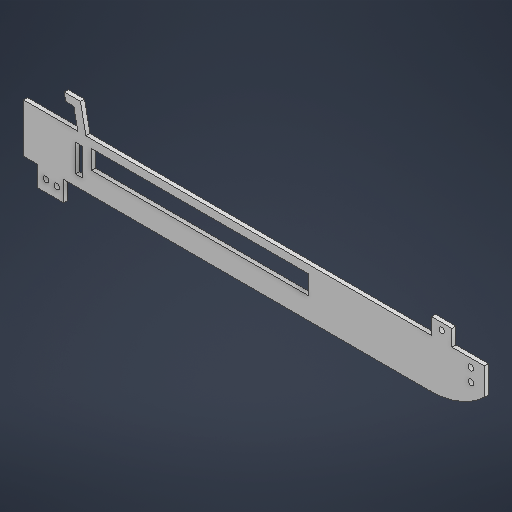
# Autodesk Inventor part: Middle_bar
Saved by Autodesk Inventor 2027 (Build 310192000, 192)
## iProperties
Created: 2026-05-09
Part Number: Middle_bar
Material: Generic
Document SubType Name: Modeling
Designer: alexy
Density: 1 g/cm^3
Appearance: Default
Mass: 26.8499 g
Surface Area: 216.911 cm^2
Volume: 26.8499 cm^3
Author: alexy
Autodesk Inventor part; units mm, degrees
ref_plane "YZ Plane" through (0, 0, 0) normal (1, 0, 0) x (0, 1, 0)
ref_plane "XZ Plane" through (0, 0, 0) normal (0, 1, 0) x (-1, 0, 0)
ref_plane "XY Plane" through (0, 0, 0) normal (0, 0, 1) x (1, 0, 0)
sketch "Sketch1" plane through (0, 0, 0) normal (0, 0, 1) x (1, 0, 0)
  line L0 (0, 0) -> (300, 0)
  line L1 (300, 0) -> (300, 16)
  line L2 (300, 16) -> (0, 16)
  line L3 (0, 16) -> (0, 0)
  line L4 (0, 0) -> (22.0483, 0)
  line L5 (10, 0) -> (29.5, 0)
  line L6 (29.5, 0) -> (29.5, -15)
  line L7 (29.5, -15) -> (10, -15)
  line L8 (10, -15) -> (10, 0)
  point P0 (0, 8)
  dimension "d2" = 19.5
  dimension "d3" = 15
  dimension "d4" = 10
  dimension "d5" = 16
  dimension "d8" = 300
  constraints: 18 end point, 4 parallel, 3 horizontal, 2 perpendicular, 1 midpoint, 1 point on line
  measures "d2" distance of L6.end L7.end
  measures "d3" distance of L5.end L6.end
  measures "d4" distance of L0.start L5.start
  measures "d5" distance of L2.end L0.start
  measures "d8" distance of L1.end L2.end
extrude "Extrusion1" add sketch "Sketch1" along normal blind 3
sketch "Sketch2" plane through (0, 0, 3) normal (0, 0, 1) x (1, 0, 0)
  line L0 (0, 16) -> (0, 0) projected
  line L1 (0, 16) -> (0, 36)
  line L2 (300, 0) -> (300, 16) projected
  line L3 (340, 16) -> (340, 36)
  line L4 (340, 36) -> (0, 36)
  line L5 (300, 16) -> (0, 16) projected
  line L6 (50, 16) -> (50, 30)
  line L7 (50, 30) -> (210, 30)
  line L8 (210, 30) -> (210, 16)
  line L9 (40, 36) -> (36, 56)
  line L10 (36, 56) -> (42, 56)
  line L11 (42, 56) -> (46, 36)
  circle A0 centre (330, 30) radius 2.1
  circle A1 centre (330, 20.6) radius 2.1
  line L12 (340, 16) -> (300, 16)
  line L13 (301, 36) -> (316, 36)
  line L14 (316, 36) -> (316, 48)
  line L15 (316, 48) -> (301, 48)
  line L16 (301, 48) -> (301, 36)
  circle A2 centre (308.5, 43) radius 2.075
  line L17 (36, 56) -> (30, 56)
  line L18 (30, 56) -> (31.1, 50.5)
  line L19 (31.1, 50.5) -> (37.1, 50.5)
  point P0 (308.5, 48)
  point P1 (316, 36)
  dimension "d44" = 20
  dimension "d45" = 160
  dimension "d46" = 50
  dimension "d47" = 14
  dimension "d48" = 20
  dimension "d49" = 6
  dimension "d50" = 4
  dimension "d51" = 40
  dimension "d83" = 4.2
  dimension "d84" = 4.2
  dimension "d85" = 6
  dimension "d86" = 9.4
  dimension "d87" = 10
  dimension "d99" = 40
  dimension "d107" = 7
  dimension "d108" = 15
  dimension "d109" = 12
  dimension "d110" = 24
  dimension "d111" = 4.15
  dimension "d112" = 6
  dimension "d114" = 5.5
  constraints: 34 end point, 6 parallel, 6 point on line, 5 perpendicular, 3 centre point, 3 horizontal, 3 vertical alignment, 1 midpoint, 1 vertical
  measures "d44" distance of L0.start L1.end
  measures "d45" distance of L6.end L7.end
  measures "d46" distance between parallel lines of L1 L6
  measures "d47" distance of L6.start L6.end
  measures "d48" distance between parallel lines of L4 L10
  measures "d49" distance of L9.end L10.end
  measures "d50" horizontal distance of L9.start L9.end
  measures "d51" distance of L1.end L9.start
  measures "d83" diameter of A0
  measures "d84" diameter of A1
  measures "d85" distance from line of L4 A0.centre
  measures "d86" distance of A1.centre A0.centre
  measures "d87" distance from line of L3 A0.centre
  measures "d99" distance of L3.start L2.end
  measures "d107" distance from line of L4 A2.centre
  measures "d108" distance of L14.end L15.end
  measures "d109" distance of L13.end L14.end
  measures "d110" distance of L13.end L3.end
  measures "d111" diameter of A2
  measures "d112" distance of L9.end L17.end
  measures "d114" vertical distance of L17.end L18.end
extrude "Extrusion2" add sketch "Sketch2" against normal blind 3 contours L1 L4 L3 L12 L5 L8 L7 L6 | L9 L10 L11 L4 | L19 L18 L17 L9 | L16 L15 L14 L4
sketch "Sketch3" plane through (0, 0, 3) normal (0, 0, 1) x (1, 0, 0)
  circle A0 centre (16.5, -6.5) radius 2.1
  circle A1 centre (24.5, -7) radius 2.1
  line L0 (29.5, 0) -> (300, 0) projected
  line L1 (29.5, -15) -> (29.5, 0) projected
  point P0 (0, 0)
  dimension "d75" = 4.2
  dimension "d76" = 6.5
  dimension "d77" = 4.2
  dimension "d78" = 7
  dimension "d79" = 5
  dimension "d80" = 8
  constraints: 2 centre point
  measures "d75" diameter of A0
  measures "d76" vertical distance of point (0, 0) A0.centre
  measures "d77" diameter of A1
  measures "d78" distance from line of L0 A1.centre
  measures "d79" distance from line of L1 A1.centre
  measures "d80" horizontal distance of A1.centre A0.centre
extrude "Extrusion3" cut sketch "Sketch3" against normal blind 3
sketch "Sketch4" plane through (0, 0, 3) normal (0, 0, 1) x (1, 0, 0)
  line L0 (29.5, 0) -> (300, 0) projected
  circle A0 centre (41, 18) radius 2.6
  line L1 (340, 36) -> (46, 36) projected
  line L2 (38.4, 28.1) -> (43.6, 28.1)
  line L3 (43.6, 28.1) -> (43.6, 7.9)
  line L4 (43.6, 7.9) -> (38.4, 7.9)
  line L5 (38.4, 7.9) -> (38.4, 28.1)
  line L6 (38.4, 28.1) -> (43.6, 7.9) construction
  line L7 (43.6, 28.1) -> (38.4, 7.9) construction
  point P0 (0, 0)
  point P1 (43.6, 18)
  point P2 (38.4, 18)
  dimension "d95" = 18
  dimension "d96" = 5.2
  dimension "d100" = 5
  dimension "d101" = 20.2
  constraints: 12 end point, 2 midpoint, 2 parallel, 1 centre point, 1 coincident, 1 horizontal, 1 perpendicular, 1 tangent
  measures "d95" distance from line of L1 A0.centre
  measures "d96" diameter of A0
  measures "d100" horizontal distance of A0.centre L1.end
  measures "d101" distance of L2.end L3.end
extrude "Extrusion4" cut sketch "Sketch4" against normal blind 3
sketch "Sketch5" plane through (0, 0, 3) normal (0, 0, 1) x (1, 0, 0)
  line L0 (29.5, 0) -> (300, 0) projected
  line L1 (340, 36) -> (340, 16) projected
  arc A0 (300, 0) -> (340, 16) centre (300, 58) ccw
  line L2 (300, 0) -> (300, 16) projected
  line L3 (300, 0) -> (300, 16)
  line L4 (300, 16) -> (340, 16)
  point P0 (0, 0)
  constraints: 4 end point, 2 point on circle, 1 centre point, 1 collinear, 1 perpendicular, 1 tangent
extrude "Extrusion5" add sketch "Sketch5" against normal blind 3
body "Solid1"
